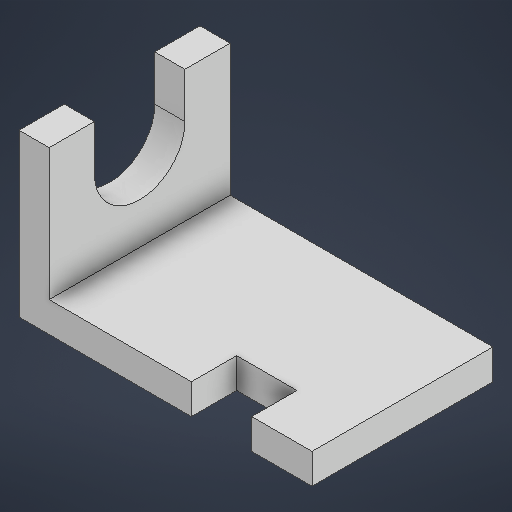
# Autodesk Inventor part: Part11
Saved by Autodesk Inventor 2026.2 (Build 302298000, 298)
## iProperties
Created: 2026-05-04
Part Number: Part11
Material: Generic
Document SubType Name: Modeling
Designer: LENOVO
Density: 1 g/cm^3
Appearance: Default
Author: LENOVO
Autodesk Inventor part; units mm, degrees
ref_plane "YZ Plane" through (0, 0, 0) normal (1, 0, 0) x (0, 1, 0)
ref_plane "XZ Plane" through (0, 0, 0) normal (0, 1, 0) x (-1, 0, 0)
ref_plane "XY Plane" through (0, 0, 0) normal (0, 0, 1) x (1, 0, 0)
sketch "Sketch1" plane through (0, 0, 0) normal (0, 0, 1) x (1, 0, 0)
  line L0 (-47.0946, 30.5405) -> (-47.0946, -23.1081)
  line L1 (-47.0946, -23.1081) -> (50.0676, -23.1081)
  line L2 (50.0676, -23.1081) -> (50.0676, -13.1081)
  line L3 (50.0676, -13.1081) -> (-37.0946, -13.1081)
  line L4 (-37.0946, -13.1081) -> (-37.0946, 30.5405)
  line L5 (-37.0946, 30.5405) -> (-47.0946, 30.5405)
  point P0 (0, 0)
  dimension "d0" = 10
  dimension "d1" = 10
  constraints: 12 end point, 5 perpendicular, 1 vertical
  measures "d0" distance of L4.end L0.start
  measures "d1" distance of L1.end L2.end
extrude "Extrusion1" add sketch "Sketch1" against normal blind 60
sketch "Sketch2" plane through (-47.0946, -23.1081, 0) normal (-1, 0, 0) x (0, 0, 1)
  line L0 (-60, 0) -> (-60, 53.6486) projected
  line L1 (0, 53.6486) -> (-60, 53.6486) projected
  line L2 (-45, 53.6486) -> (-45, 23.6486)
  line L3 (-45, 23.6486) -> (-15, 23.6486)
  line L4 (-15, 23.6486) -> (-15, 53.6486)
  point P0 (0, 23.1081)
  dimension "d4" = 15
  dimension "d5" = 15
  dimension "d6" = 30
  dimension "d7" = 30
  constraints: 6 end point, 2 perpendicular, 2 point on line, 1 coincident, 1 vertical
  measures "d4" distance of L0.end L2.start
  measures "d5" distance of L1.start L4.end
  measures "d6" distance of L4.end L2.start
  measures "d7" distance of L3.end L4.end
extrude "Extrusion2" cut sketch "Sketch2" against normal blind 40
fillet "Fillet1" radius 15 2 edges at (-42.0946, 0.5405, -45) (-42.0946, 0.5405, -15)
sketch "Sketch3" plane through (-37.0946, -13.1081, 0) normal (0, 1, 0) x (1, 0, 0)
  line L0 (-10, 0) -> (87.1622, 0) projected
  line L1 (47.1622, 0) -> (47.1622, 15)
  line L2 (47.1622, 15) -> (67.1622, 15)
  line L3 (67.1622, 15) -> (67.1622, 0)
  point P0 (37.0946, 0)
  dimension "d11" = 20
  dimension "d12" = 20
  dimension "d13" = 15
  constraints: 6 end point, 2 perpendicular, 2 point on line, 1 vertical
  measures "d11" distance of L0.end L3.end
  measures "d12" distance of L3.end L1.start
  measures "d13" distance of L1.start L1.end
extrude "Extrusion3" cut sketch "Sketch3" against normal through all
body "Solid1"
